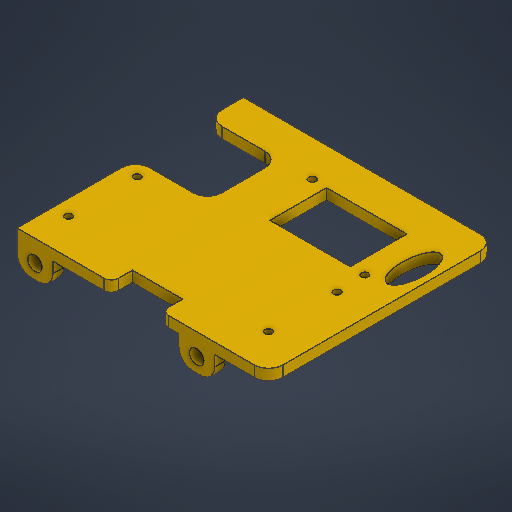
# Autodesk Inventor part: servo_driver_support
Saved by Autodesk Inventor 2026.1 (Build 301233000, 233)
## iProperties
Created: 2026-04-24
Part Number: servo_driver_support
Material: Generic
Document SubType Name: Modeling
Designer: emanuel
Density: 1 g/cm^3
Appearance: Default
Author: emanuel
Autodesk Inventor part; units mm, degrees
ref_plane "YZ Plane" through (0, 0, 0) normal (1, 0, 0) x (0, 1, 0)
ref_plane "XZ Plane" through (0, 0, 0) normal (0, 1, 0) x (-1, 0, 0)
ref_plane "XY Plane" through (0, 0, 0) normal (0, 0, 1) x (1, 0, 0)
sketch "Sketch1" plane through (0, 0, 0) normal (0, 1, 0) x (-1, 0, 0)
  line L0 (0, 0) -> (55, 0)
  line L1 (55, 0) -> (55, -63)
  line L2 (55, -63) -> (0, -63)
  line L3 (0, -63) -> (0, 0)
  dimension "d0" = 55
  dimension "d1" = 63
  constraints: 8 end point, 2 parallel, 1 horizontal, 1 perpendicular
  measures "d0" distance of L1.end L2.end
  measures "d1" distance of L0.end L1.end
extrude "Extrusion1" add sketch "Sketch1" along normal blind 3
sketch "Sketch2" plane through (0, 0, 0) normal (0, -1, 0) x (1, 0, 0)
  line L0 (0, 0) -> (-10, 0)
  line L1 (-10, 0) -> (-10, -3)
  line L2 (-10, -3) -> (0, -3)
  line L3 (0, -3) -> (0, 0)
  line L4 (-55, -63) -> (-55, 0) projected
  line L5 (-55, 0) -> (-45, 0)
  line L6 (-45, 0) -> (-45, -3)
  line L7 (-45, -3) -> (-55, -3)
  line L8 (-55, -3) -> (-55, 0)
  line L9 (-55, -63) -> (-45, -63)
  line L10 (-45, -63) -> (-45, -60)
  line L11 (-45, -60) -> (-55, -60)
  line L12 (-55, -60) -> (-55, -63)
  line L13 (0, -63) -> (-10, -63)
  line L14 (-10, -63) -> (-10, -60)
  line L15 (-10, -60) -> (0, -60)
  line L16 (0, -60) -> (0, -63)
  dimension "d4" = 10
  dimension "d5" = 3
  dimension "d6" = 10
  dimension "d7" = 3
  dimension "d8" = 10
  dimension "d9" = 3
  dimension "d10" = 10
  dimension "d11" = 3
  constraints: 32 end point, 8 parallel, 4 horizontal, 4 perpendicular, 2 point on line
  measures "d4" distance of L2.end L1.end
  measures "d5" distance of L1.end L0.end
  measures "d6" distance of L6.end L7.end
  measures "d7" distance of L5.end L6.end
  measures "d8" distance of L11.end L10.end
  measures "d9" distance of L10.end L9.end
  measures "d10" distance of L14.end L15.end
  measures "d11" distance of L13.end L14.end
extrude "Extrusion2" add sketch "Sketch2" along normal blind 7
sketch "Sketch3" plane through (-55, 3, 0) normal (0, 0, 1) x (1, 0, 0)
  line L0 (10, -10) -> (0, -10) projected
  line L1 (0, -10) -> (5, -10)
  line L2 (5, -10) -> (5, -6)
  line L3 (5, -6) -> (0, -6)
  line L4 (0, -6) -> (0, -10)
  line L5 (45, -3) -> (45, -10) projected
  line L6 (45, -10) -> (50, -10)
  line L7 (50, -10) -> (50, -6)
  line L8 (50, -6) -> (45, -6)
  line L9 (45, -6) -> (45, -10)
  circle A0 centre (5, -6) radius 2
  circle A1 centre (50, -6) radius 2
  point P0 (55, -3)
  dimension "d14" = 5
  dimension "d15" = 4
  dimension "d16" = 5
  dimension "d17" = 4
  dimension "d18" = 4
  dimension "d19" = 4
  constraints: 16 end point, 4 parallel, 2 centre point, 2 coincident, 2 horizontal, 2 perpendicular
  measures "d14" distance of L3.end L2.end
  measures "d15" distance of L2.end L1.end
  measures "d16" distance of L8.end L7.end
  measures "d17" distance of L7.end L6.end
  measures "d18" diameter of A0
  measures "d19" diameter of A1
extrude "Extrusion3" cut sketch "Sketch3" against normal up to surface (63 mm away) contours A0 L3 L2 | L2 L3 A0 | A1 L7 L8 | L8 L7 A1
fillet "Fillet1" radius 4 8 edges at (0, -7, -1.5) (-10, -7, -61.5) (0, -7, -61.5) (-45, -7, -61.5) (-55, -7, -61.5) (-45, -7, -1.5) (-55, -7, -1.5) (-10, -7, -1.5)
sketch "Sketch4" plane through (0, 3, 0) normal (0, 1, 0) x (1, 0, 0)
  line L0 (0, 0) -> (15, 0)
  line L1 (15, 0) -> (15, 63)
  line L2 (15, 63) -> (0, 63)
  line L3 (0, 63) -> (0, 0)
  dimension "d23" = 15
  dimension "d24" = 63
  constraints: 8 end point, 2 parallel, 1 horizontal, 1 perpendicular
  measures "d23" distance of L2.end L1.end
  measures "d24" distance of L0.end L1.end
extrude "Extrusion4" add sketch "Sketch4" against normal blind 3
sketch "Sketch5" plane through (0, 3, 0) normal (0, 1, 0) x (1, 0, 0)
  line L0 (14.6866, 62.7723) -> (4.6866, 62.7723)
  line L1 (4.6866, 62.7723) -> (4.6866, 52.7723)
  line L2 (4.6866, 52.7723) -> (14.6866, 52.7723)
  line L3 (14.6866, 52.7723) -> (14.6866, 62.7723)
  line L4 (4.6866, 52.7723) -> (-25.6434, 52.7723)
  line L5 (-25.6434, 52.7723) -> (-25.6434, 37.0423)
  line L6 (-25.6434, 37.0423) -> (4.6866, 37.0423)
  line L7 (4.6866, 37.0423) -> (4.6866, 52.7723)
  circle A0 centre (-25.6434, 52.7723) radius 1
  circle A1 centre (4.6866, 37.0423) radius 1
  circle A2 centre (4.6866, 37.0423) radius 2
  circle A3 centre (-25.6434, 52.7723) radius 2
  point P0 (0, 0)
  dimension "d27" = 10
  dimension "d28" = 10
  dimension "d29" = 30.33
  dimension "d30" = 15.73
  dimension "d31" = 2
  dimension "d32" = 2
  dimension "d33" = 4
  dimension "d34" = 4
  constraints: 16 end point, 4 centre point, 4 coincident, 4 parallel, 2 horizontal, 2 perpendicular
  measures "d27" distance of L2.end L1.end
  measures "d28" distance of L1.end L0.end
  measures "d29" distance of L6.end L5.end
  measures "d30" distance of L5.end L4.end
  measures "d31" diameter of A0
  measures "d32" diameter of A1
  measures "d33" diameter of A2
  measures "d34" diameter of A3
extrude "Extrusion5" cut sketch "Sketch5" against normal blind 3 contours A0 L5 L4 | L4 L5 A0 | A1 L6 L7 | L7 L6 A1
sketch "Sketch6" plane through (0, 3, 0) normal (0, 1, 0) x (1, 0, 0)
  line L0 (15, 63) -> (-55, 63) projected
  line L1 (-55, 63) -> (-55, 53)
  line L2 (-55, 53) -> (-35, 53)
  line L3 (-35, 53) -> (-35, 33)
  line L4 (-35, 33) -> (-55, 33)
  line L5 (-55, 33) -> (-55, 53)
  point P0 (0, 0)
  dimension "d37" = 10
  dimension "d38" = 20
  dimension "d39" = 20
  constraints: 10 end point, 2 parallel, 1 horizontal, 1 perpendicular, 1 vertical
  measures "d37" distance of L0.end L1.end
  measures "d38" distance of L3.end L4.end
  measures "d39" distance of L2.end L3.end
extrude "Extrusion6" cut sketch "Sketch6" against normal blind 3
fillet "Fillet2" radius 4 4 edges at (-35, 1.5, -53) (-35, 1.5, -33) (-55, 1.5, -53) (-55, 1.5, -33)
fillet "Fillet3" radius 4 2 edges at (15, 1.5, 0) (15, 1.5, -63)
sketch "Sketch7" plane through (0, 3, 0) normal (0, 1, 0) x (1, 0, 0)
  line L0 (15, 0) -> (5, 0)
  line L1 (5, 0) -> (5, 10)
  line L2 (5, 10) -> (15, 10)
  line L3 (15, 10) -> (15, 0)
  line L4 (5, 10) -> (-50.626, 10)
  line L5 (-50.626, 10) -> (-50.626, 16.3068)
  line L6 (5, 16.3068) -> (5, 10)
  line L7 (5, 10) -> (-50.626, 10)
  line L8 (-50.626, 10) -> (-50.626, 29.05)
  line L9 (-50.626, 29.05) -> (5, 29.05)
  line L10 (5, 29.05) -> (5, 10)
  circle A0 centre (-50.626, 10) radius 1
  circle A1 centre (-50.626, 29.05) radius 1
  circle A2 centre (5, 29.05) radius 1
  circle A3 centre (5, 10) radius 1
  point P0 (0, 0)
  dimension "d44" = 10
  dimension "d45" = 10
  dimension "d48" = 55.626
  dimension "d49" = 19.05
  dimension "d50" = 2
  dimension "d51" = 2
  dimension "d52" = 2
  dimension "d53" = 2
  constraints: 22 end point, 5 parallel, 4 centre point, 4 coincident, 3 horizontal, 3 perpendicular
  measures "d44" distance of L1.end L2.end
  measures "d45" distance of L0.end L1.end
  measures "d48" distance of L8.end L9.end
  measures "d49" distance of L7.end L8.end
  measures "d50" diameter of A0
  measures "d51" diameter of A1
  measures "d52" diameter of A2
  measures "d53" diameter of A3
extrude "Extrusion7" cut sketch "Sketch7" against normal blind 3 contours A3 L4 L1 | L1 L2 A3 | L2 L6 A3 | L4 A3 L6 | A0 L5 L4 | L4 L5 A0 | A2 L9 L10 | L10 L9 A2 | A1 L9 L8 | L8 L9 A1
sketch "Sketch8" plane through (0, 3, 0) normal (0, 1, 0) x (1, 0, 0)
  circle A0 centre (-25.6434, 52.7723) radius 1 projected
  line L0 (-25.6434, 52.7723) -> (-21.6434, 52.7723)
  circle A1 centre (4.6866, 37.0423) radius 1 projected
  line L1 (4.6866, 37.0423) -> (0.6866, 37.0423)
  line L2 (-21.6434, 52.7723) -> (0.6866, 52.7723)
  line L3 (0.6866, 52.7723) -> (0.6866, 37.0423)
  line L4 (0.6866, 37.0423) -> (-21.6434, 37.0423)
  line L5 (-21.6434, 37.0423) -> (-21.6434, 52.7723)
  point P0 (0, 0)
  dimension "d56" = 4
  dimension "d57" = 4
  constraints: 12 end point, 3 horizontal, 2 parallel, 1 perpendicular
  measures "d56" distance of L0.start L0.end
  measures "d57" distance of L1.start L1.end
extrude "Extrusion8" cut sketch "Sketch8" against normal blind 10 contours L2 L3 L4 L5
sketch "Sketch9" plane through (0, 3, 0) normal (0, 1, 0) x (1, 0, 0)
  line L0 (-28.7673, 5.8913) -> (-14.8119, 5.8913)
  line L1 (-14.8119, 5.8913) -> (-14.8119, -0.376)
  line L2 (-14.8119, -0.376) -> (-28.7673, -0.376)
  line L3 (-28.7673, -0.376) -> (-28.7673, 5.8913)
  point P0 (0, 0)
  constraints: 8 end point, 2 parallel, 1 horizontal, 1 perpendicular
extrude "Extrusion9" cut sketch "Sketch9" against normal blind 10
fillet "Fillet4" radius 2 2 edges at (-28.7673, 1.5, 0) (-14.8119, 1.5, 0)
sketch "Sketch10" plane through (0, 3, 0) normal (0, 1, 0) x (1, 0, 0)
  ellipse E0 centre (9.9899, 45.4239) end of major axis (9.9899, 52.7522) minor radius 3.154
  point P0 (0, 0)
  constraints: 2 other
extrude "Extrusion10" cut sketch "Sketch10" against normal blind 10
body "Solid1"
